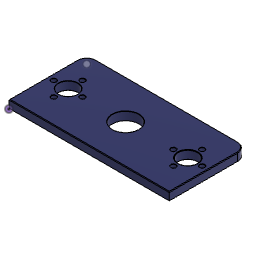
Bearing Bracket v3 (Autodesk Fusion 360 design; units mm, degrees)
Autodesk Fusion 360 part; units mm, degrees
sketch "Sketch1" plane through (0, 0, 7) normal (0, 0, 1) x (-1, 0, 0)
sketch "Sketch2" plane through (0, 0, 0) normal (0, 0, 1) x (1, 0, 0) in component "Bearing Bracket"
  point P0 (0, 65)
  dimension "d2" = 65
  measures "d2" distance of origin P0
sketch "Sketch3" plane through (0, 0, 7) normal (0, 0, 1) x (-1, 0, 0) in component "Bearing Bracket"
  circle A0 centre (-17, -32.5) radius 4
  circle A1 centre (-64.9939, -32.5034) radius 11
  circle A2 centre (-117, -32.5) radius 4
  arc A3 (-134, -57) -> (-126, -65) centre (-126, -57) ccw
  line L0 (-126, -65) -> (-8, -65)
  arc A4 (-8, -65) -> (0, -57) centre (-8, -57) ccw
  line L1 (0, -57) -> (0, 0)
  line L2 (0, 0) -> (-134, 0)
  line L3 (-134, 0) -> (-134, -57)
  circle A5 centre (-64.9939, -32.5034) radius 10.5
  dimension "d3" = -0.5
extrude "Extrude1" add sketch "Sketch3" against normal blind 7 contours A3 L0 A4 L1 L2 L3
chamfer "Chamfer1" distance 0.2 angle 45 3 edges at (120.7293, 31.0535, 7) (75.2495, 28.5256, 7) (20.7293, 31.0535, 7)
chamfer "Chamfer2" distance 0.2 angle 45 1 edges at (20.7293, 33.9465, 0)
chamfer "Chamfer3" distance 0.2 angle 45 1 edges at (120.7293, 33.9465, 0)
chamfer "Chamfer4" distance 0.5 angle 45 6 edges at (134, 28.5, 0) (0, 28.5, 0) (2.3431, 62.6569, 0) (67, 65, 0) (131.6569, 62.6569, 0) (67, 0, 0)
chamfer "Chamfer5" distance 0.5 angle 45 6 edges at (0, 28.5, 7) (134, 28.5, 7) (131.6569, 62.6569, 7) (67, 65, 7) (2.3431, 62.6569, 7) (67, 0, 7)
sketch "Sketch2 (2)" plane through (0, 0, 7) normal (0, 0, 1) x (-1, 0, 0)
  circle A0 centre (-17, -32.5) radius 4.2
  circle A1 centre (-117, -32.5) radius 4.2
  circle A2 centre (-64.9939, -32.5034) radius 11.2
  line L0 (-133.5, -0.5) -> (-133.5, -57)
  arc A3 (-133.5, -57) -> (-126, -64.5) centre (-126, -57) ccw
  line L1 (-126, -64.5) -> (-8, -64.5)
  arc A4 (-8, -64.5) -> (-0.5, -57) centre (-8, -57) ccw
  line L2 (-0.5, -57) -> (-0.5, -0.5)
  line L3 (-0.5, -0.5) -> (-133.5, -0.5)
  circle A5 centre (-17, -32.5) radius 8
  circle A6 centre (-117, -32.5) radius 8
  line L4 (-117, -32.5) -> (-117, -44.5)
  line L5 (-117, -32.5) -> (-117, -20.5)
  line L6 (-117, -32.5) -> (-105, -32.5)
  line L7 (-117, -32.5) -> (-129, -32.5)
  circle A7 centre (-117, -44.5) radius 2
  circle A8 centre (-129, -32.5) radius 2
  circle A9 centre (-117, -20.5) radius 2
  circle A10 centre (-105, -32.5) radius 2
  line L8 (-17, -32.5) -> (-17, -44.5)
  line L9 (-17, -32.5) -> (-17, -20.5)
  line L10 (-17, -32.5) -> (-29, -32.5)
  line L11 (-17, -32.5) -> (-5, -32.5)
  circle A11 centre (-17, -44.5) radius 2
  circle A12 centre (-17, -20.5) radius 2
  circle A13 centre (-29, -32.5) radius 2
  circle A14 centre (-5, -32.5) radius 2
  dimension "d11" = 16
  dimension "d12" = 16
  dimension "d13" = 12
  dimension "d14" = 12
  dimension "d15" = 12
  dimension "d16" = 12
  dimension "d17" = 4
  dimension "d18" = 4
  dimension "d19" = 4
  dimension "d20" = 4
  dimension "d21" = 12
  dimension "d22" = 12
  dimension "d23" = 12
  dimension "d24" = 12
  dimension "d25" = 4
  dimension "d26" = 4
  dimension "d27" = 4
  dimension "d28" = 4
  constraint concentric A0 A5
  constraint concentric A1 A6
  constraint coincident A1.centre A6.centre
  constraint vertical L4
  constraint parallel L4 L5
  constraint perpendicular L4 L6
  constraint perpendicular L4 L7
  constraint coincident L4.end A7.centre
  constraint coincident L7.end A8.centre
  constraint coincident L5.end A9.centre
  constraint coincident L6.end A10.centre
  constraint coincident A0.centre A5.centre
  constraint parallel L2 L8
  constraint parallel L8 L9
  constraint perpendicular L8 L10
  constraint perpendicular L8 L11
  constraint coincident L8.end A11.centre
  constraint coincident L9.end A12.centre
  constraint coincident L10.end A13.centre
  constraint coincident L11.end A14.centre
  measures "d11" diameter of A5
  measures "d12" diameter of A6
  measures "d13" distance of A1.centre L4.end
  measures "d14" distance of A1.centre L5.end
  measures "d15" distance of A1.centre L6.end
  measures "d16" distance of A1.centre L7.end
  measures "d17" diameter of A7
  measures "d18" diameter of A8
  measures "d19" diameter of A9
  measures "d20" diameter of A10
  measures "d21" distance of A0.centre L8.end
  measures "d22" distance of A0.centre L9.end
  measures "d23" distance of A0.centre L10.end
  measures "d24" distance of A0.centre L11.end
  measures "d25" diameter of A11
  measures "d26" diameter of A12
  measures "d27" diameter of A13
  measures "d28" diameter of A14
extrude "Extrude2" cut sketch "Sketch2 (2)" against normal blind 25 contours A0 L9 L11 | A0 A5 L8 L11 | A0 L8 L11 | A0 A5 L9 L11 | A0 L9 L10 | A0 A5 L9 L10 | A0 A5 L8 L10 | A0 L8 L10 | A1 L5 L6 | A1 A6 L4 L6 | A1 L4 L6 | A1 A6 L5 L6 | A1 L5 L7 | A1 A6 L5 L7 | A1 A6 L4 L7 | A1 L4 L7 | A7 | A8 | A9 | A10 | A11 | A12 | A13 | A14
chamfer "Chamfer6" distance 0.3 angle 45 1 edges at (124.4586, 29.6071, 7)
chamfer "Chamfer7" distance 0.2 angle 45 1 edges at (118.8647, 43.7768, 7)
chamfer "Chamfer8" distance 0.2 angle 45 1 edges at (124.7383, 35.5014, 7)
chamfer "Chamfer9" distance 0.2 angle 45 1 edges at (130.8647, 31.7768, 7)
chamfer "Chamfer10" distance 0.2 angle 45 1 edges at (118.8647, 19.7768, 7)
chamfer "Chamfer11" distance 0.2 angle 45 1 edges at (106.8647, 31.7768, 7)
chamfer "Chamfer12" distance 0.2 angle 45 5 edges at (24.4586, 29.6071, 7) (30.8647, 31.7768, 7) (18.8647, 43.7768, 7) (6.8647, 31.7768, 7) (18.8647, 19.7768, 7)
chamfer "Chamfer13" distance 0.2 angle 45 10 edges at (24.4586, 35.3929, 0) (6.8647, 33.2232, 0) (18.8647, 45.2232, 0) (30.8647, 33.2232, 0) (18.8647, 21.2232, 0) (118.8647, 21.2232, 0) (124.4586, 35.3929, 0) (106.8647, 33.2232, 0) (118.8647, 45.2232, 0) (130.8647, 33.2232, 0)
component "Bearing Bracket" placed x (1, 0, 0) y (0, 1, 0) z (0, 0, 1) at (0, 0, 0)
